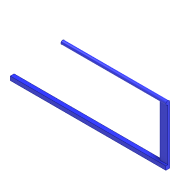
# Autodesk Inventor part: Bone17_16_Fix
Saved by Autodesk Inventor 2020 (Build 240168000, 168)
## iProperties
Created: 2021-03-17
Part Number: Bone17_16_Fix
Material: Generic
Document SubType Name: Modeling
Designer: deox
Density: 1 g/cm^3
Appearance: Blue - Wall Paint - Glossy
Author: deox
Autodesk Inventor part; units mm, degrees
ref_plane "YZ Plane" through (0, 0, 0) normal (1, 0, 0) x (0, 1, 0)
ref_plane "XZ Plane" through (0, 0, 0) normal (0, 1, 0) x (-1, 0, 0)
ref_plane "XY Plane" through (0, 0, 0) normal (0, 0, 1) x (1, 0, 0)
sketch "Sketch1" plane through (0, 0, 0) normal (1, 0, 0) x (0, 1, 0)
  circle A0 centre (0, 0) radius 0.05
  line L0 (0, 0) -> (-1.428, 0)
  line L1 (-1.478, 0.05) -> (-1.378, 0.05)
  line L2 (-1.378, 0.05) -> (-1.378, -0.05)
  line L3 (-1.378, -0.05) -> (-1.478, -0.05)
  line L4 (-1.478, -0.05) -> (-1.478, 0.05)
  line L5 (-1.478, 0.05) -> (-1.378, -0.05) construction
  line L6 (-1.378, 0.05) -> (-1.478, -0.05) construction
  line L7 (-1.378, -0.05) -> (0, -0.05)
  point P0 (-0.05, 0)
  point P1 (-1.378, 0)
  dimension "d0" = 0.1
  dimension "d1" = 1.428
  dimension "d2" = 0.1
  dimension "d3" = 0.1
  constraints: 16 end point, 2 horizontal, 2 midpoint, 2 parallel, 1 coincident, 1 perpendicular, 1 point on line, 3 other
  measures "d1" distance of L0.start L0.end
  measures "d2" distance of L2.end L3.end
  measures "d3" distance of L1.end L2.end
extrude "Extrusion1" add sketch "Sketch1" along normal blind 0.2
sketch "Sketch2" plane through (0, 0, 0) normal (-1, 0, 0) x (0, 0, 1)
  arc A0 (0, -0.05) -> (-0.05, 0) centre (0, 0) ccw projected
  circle A1 centre (0, 0) radius 0.05
  point P0 (-0.05, 0)
  point P1 (0, -0.05)
  dimension "d6" = 0.1
  constraints: 1 centre point, 1 coincident
  measures "d6" diameter of A1
extrude "Extrusion2" add sketch "Sketch2" along normal blind 2.5
sketch "Sketch3" plane through (0, 0, 0) normal (-1, 0, 0) x (0, 0, 1)
  line L0 (-0.05, -1.478) -> (-0.05, 0) projected
  line L1 (0.05, -1.478) -> (-0.05, -1.478) projected
  line L2 (-0.05, -1.478) -> (0.05, -1.478)
  line L3 (0, -1.378) -> (0.05, -1.378) projected
  line L4 (0.05, -1.478) -> (0.05, -1.378)
  line L5 (0.05, -1.378) -> (-0.05, -1.378)
  line L6 (-0.05, -1.378) -> (-0.05, -1.478)
  point P0 (0, 0)
  constraints: 8 end point, 3 perpendicular, 1 collinear, 1 point on line
extrude "Extrusion3" add sketch "Sketch3" along normal blind 3.8
body "Solid1"
